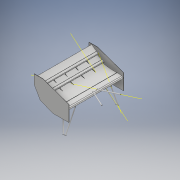
# Autodesk Inventor part: simpleRrwing
Saved by Autodesk Inventor 2018.2 (Build 222227000, 227)
## iProperties
Created: 2018-05-20
Part Number: simpleRrwing
Material: 一般
Document SubType Name: Modeling
Designer: ku_sk
Density: 1 g/cm^3
Appearance: 既定
Author: ku_sk
Autodesk Inventor part; units mm, degrees
ref_plane "YZ Plane" through (0, 0, 0) normal (1, 0, 0) x (0, 1, 0)
ref_plane "XZ Plane" through (0, 0, 0) normal (0, 1, 0) x (-1, 0, 0)
ref_plane "XY Plane" through (0, 0, 0) normal (0, 0, 1) x (1, 0, 0)
ref_plane "作業平面7" through (-254.1154, 478, -190) normal (0, 1, 0) x (1, 0, 0)
sketch "スケッチ4" plane through (-254.1154, 478, -190) normal (0, 1, 0) x (1, 0, 0)
  line L0 (-220, -86.6025) -> (0, 0) projected
  line L1 (-220, -86.6025) -> (-325.8846, -270) projected
  line L2 (-325.8846, -270) -> (-325.8846, -430) projected
  line L3 (-325.8846, -430) -> (-175.8846, -430) projected
  line L4 (-175.8846, -430) -> (274.1154, -270) projected
  line L5 (274.1154, -270) -> (274.1154, 0) projected
  line L6 (274.1154, 0) -> (0, 0) projected
  circle A0 centre (-165.8846, -335) radius 2.5 projected
  circle A1 centre (-65.8846, -265) radius 2.5 projected
  circle A2 centre (254.1154, -190) radius 2.5 projected
  point P0 (254.1154, -190)
extrude "押し出し1" add sketch "スケッチ4" against normal blind 5 contours L0 L6 L5 L4 L3 L2 L1 | A0 | A1 | A2
ref_plane "作業平面8" through (-254.1154, 473, -190) normal (0, -1, 0) x (1, 0, 0)
sketch "スケッチ5" plane through (-254.1154, 473, -190) normal (0, -1, 0) x (1, 0, 0)
  arc A0 (-98.825, 235.4012) -> (58.0734, 177.1204) centre (363.8757, 1240.7077) ccw projected
  arc A1 (-96.151, 242.9074) -> (-98.825, 235.4012) centre (-97.1526, 239.0348) ccw projected
  arc A2 (-96.151, 242.9074) -> (158.3312, 216.8528) centre (116.6772, 1065.8316) ccw projected
  arc A3 (158.3312, 216.8528) -> (163.3213, 217.108) centre (99.5256, 1415.411) ccw projected
  arc A4 (242.3807, 210.8189) -> (163.3213, 217.108) centre (179.2702, -82.4677) ccw projected
  arc A5 (262.2344, 202.6128) -> (242.3807, 210.8189) centre (229.7586, 152.1616) ccw projected
  arc A6 (263.5157, 178.3109) -> (262.2344, 202.6128) centre (254.1154, 190) ccw projected
  arc A7 (246.2233, 168.6632) -> (263.5157, 178.3109) centre (226.4942, 224.3463) ccw projected
  arc A8 (191.5251, 157.8735) -> (246.2233, 168.6632) centre (182.1223, 349.5809) ccw projected
  arc A9 (103.8035, 165.4256) -> (191.5251, 157.8735) centre (175.4883, 484.8376) ccw projected
  arc A10 (58.0734, 177.1204) -> (103.8035, 165.4256) centre (278.4325, 943.5344) ccw projected
  arc A11 (-197.55, 319.0808) -> (-142.9628, 280.3195) centre (85.3008, 659.5991) ccw projected
  arc A12 (-195.7398, 321.7041) -> (-197.55, 319.0808) centre (-196.5276, 320.3115) ccw projected
  arc A13 (-195.7398, 321.7041) -> (-100.1128, 285.2914) centre (-28.3139, 617.624) ccw projected
  arc A14 (-100.1128, 285.2914) -> (-98.1583, 284.8734) centre (1.2504, 754.4668) ccw projected
  arc A15 (-68.2632, 274.2587) -> (-98.1583, 284.8734) centre (-123.0105, 167.4751) ccw projected
  arc A16 (-61.4419, 269.0327) -> (-68.2632, 274.2587) centre (-79.2127, 252.902) ccw projected
  arc A17 (-63.4627, 259.5105) -> (-61.4419, 269.0327) centre (-65.8846, 265) ccw projected
  arc A18 (-71.1428, 257.5731) -> (-63.4627, 259.5105) centre (-73.0008, 281.13) ccw projected
  arc A19 (-93.3936, 259.0671) -> (-71.1428, 257.5731) centre (-77.1795, 334.1106) ccw projected
  arc A20 (-126.5048, 271.0666) -> (-93.3936, 259.0671) centre (-65.7399, 387.0566) ccw projected
  arc A21 (-142.9628, 280.3195) -> (-126.5048, 271.0666) centre (21.5225, 553.6259) ccw projected
  arc A22 (-279.0665, 421.3155) -> (-236.3714, 369.7468) centre (82.279, 677.0238) ccw projected
  arc A23 (-276.6389, 423.381) -> (-279.0665, 421.3155) centre (-277.7604, 422.2398) ccw projected
  arc A24 (-276.6389, 423.381) -> (-193.6946, 363.4589) centre (-38.3283, 665.8846) ccw projected
  arc A25 (-193.6946, 363.4589) -> (-191.915, 362.5493) centre (25.6461, 790.4128) ccw projected
  arc A26 (-165.7858, 344.5588) -> (-191.915, 362.5493) centre (-246.3053, 255.5835) ccw projected
  arc A27 (-160.5495, 337.7454) -> (-165.7858, 344.5588) centre (-181.8897, 326.7638) ccw projected
  arc A28 (-164.966, 329.0707) -> (-160.5495, 337.7454) centre (-165.8846, 335) ccw projected
  arc A29 (-172.8859, 329.1871) -> (-164.966, 329.0707) centre (-168.5836, 352.4222) ccw projected
  arc A30 (-193.9918, 336.3891) -> (-172.8859, 329.1871) centre (-158.9075, 404.679) ccw projected
  arc A31 (-222.869, 356.5496) -> (-193.9918, 336.3891) centre (-134.1543, 452.8602) ccw projected
  arc A32 (-236.3714, 369.7468) -> (-222.869, 356.5496) centre (-6.754, 591.1686) ccw projected
  point P0 (254.1154, 190)
extrude "押し出し2" add sketch "スケッチ5" along normal blind 186
sketch "スケッチ6" plane through (-254.1154, 287, -190) normal (0, -1, 0) x (1, 0, 0)
  arc A0 (-197.1682, 321.7777) -> (-197.55, 319.0808) centre (-196.5276, 320.3115) ccw projected
  arc A1 (-197.55, 319.0808) -> (-142.9628, 280.3195) centre (85.3008, 659.5991) ccw projected
  arc A2 (-142.9628, 280.3195) -> (-126.5048, 271.0666) centre (21.5225, 553.6259) ccw projected
  line L0 (-126.5048, 271.0666) -> (-94.3475, 254.22) projected
  arc A3 (-93.447, 249.6278) -> (-94.3475, 254.22) centre (-95.7396, 251.5626) ccw projected
  line L1 (-93.447, 249.6278) -> (-100.2095, 241.6146) projected
  arc A4 (-100.2095, 241.6146) -> (-98.825, 235.4012) centre (-97.1526, 239.0348) ccw projected
  arc A5 (-98.825, 235.4012) -> (58.0734, 177.1204) centre (363.8757, 1240.7077) ccw projected
  arc A6 (58.0734, 177.1204) -> (103.8035, 165.4256) centre (278.4325, 943.5344) ccw projected
  arc A7 (103.8035, 165.4256) -> (191.5251, 157.8735) centre (175.4883, 484.8376) ccw projected
  arc A8 (191.5251, 157.8735) -> (246.2233, 168.6632) centre (182.1223, 349.5809) ccw projected
  arc A9 (246.2233, 168.6632) -> (263.5157, 178.3109) centre (226.4942, 224.3463) ccw projected
  arc A10 (263.5157, 178.3109) -> (262.2344, 202.6128) centre (254.1154, 190) ccw projected
  arc A11 (262.2344, 202.6128) -> (242.3807, 210.8189) centre (229.7586, 152.1616) ccw projected
  arc A12 (242.3807, 210.8189) -> (163.3213, 217.108) centre (179.2702, -82.4677) ccw projected
  arc A13 (158.3312, 216.8528) -> (163.3213, 217.108) centre (99.5256, 1415.411) ccw projected
  arc A14 (-23.7761, 227.5161) -> (158.3312, 216.8528) centre (116.6772, 1065.8316) ccw projected
  arc A15 (-33.5904, 230.2106) -> (-23.7761, 227.5161) centre (-15.5142, 276.8287) ccw projected
  line L2 (-33.5904, 230.2106) -> (-75.8322, 246.5899) projected
  arc A16 (-76.0007, 253.979) -> (-75.8322, 246.5899) centre (-74.3861, 250.3193) ccw projected
  line L3 (-76.0007, 253.979) -> (-63.4627, 259.5105) projected
  arc A17 (-63.4627, 259.5105) -> (-61.4419, 269.0327) centre (-65.8846, 265) ccw projected
  arc A18 (-61.4419, 269.0327) -> (-68.2632, 274.2587) centre (-79.2127, 252.902) ccw projected
  arc A19 (-68.2632, 274.2587) -> (-98.1583, 284.8734) centre (-123.0105, 167.4751) ccw projected
  arc A20 (-100.1128, 285.2914) -> (-98.1583, 284.8734) centre (1.2504, 754.4668) ccw projected
  arc A21 (-133.4564, 294.2897) -> (-100.1128, 285.2914) centre (-28.3139, 617.624) ccw projected
  arc A22 (-147.5202, 301.4877) -> (-133.4564, 294.2897) centre (-117.9943, 341.8389) ccw projected
  line L4 (-147.5202, 301.4877) -> (-173.8847, 320.7792) projected
  arc A23 (-172.135, 327.9601) -> (-173.8847, 320.7792) centre (-171.5226, 324.0073) ccw projected
  line L5 (-172.135, 327.9601) -> (-164.966, 329.0707) projected
  arc A24 (-164.966, 329.0707) -> (-160.5495, 337.7454) centre (-165.8846, 335) ccw projected
  arc A25 (-160.5495, 337.7454) -> (-165.7858, 344.5588) centre (-181.8897, 326.7638) ccw projected
  arc A26 (-165.7858, 344.5588) -> (-191.915, 362.5493) centre (-246.3053, 255.5835) ccw projected
  arc A27 (-193.6946, 363.4589) -> (-191.915, 362.5493) centre (25.6461, 790.4128) ccw projected
  arc A28 (-276.6389, 423.381) -> (-193.6946, 363.4589) centre (-38.3283, 665.8846) ccw projected
  arc A29 (-276.6389, 423.381) -> (-279.0665, 421.3155) centre (-277.7604, 422.2398) ccw projected
  arc A30 (-279.0665, 421.3155) -> (-236.3714, 369.7468) centre (82.279, 677.0238) ccw projected
  arc A31 (-236.3714, 369.7468) -> (-222.869, 356.5496) centre (-6.754, 591.1686) ccw projected
  line L6 (-222.869, 356.5496) -> (-192.3777, 328.463) projected
  arc A32 (-193.2092, 323.5074) -> (-192.3777, 328.463) centre (-194.4102, 326.2565) ccw projected
  line L7 (-193.2092, 323.5074) -> (-197.1682, 321.7777) projected
  point P0 (254.1154, 190)
extrude "押し出し3" add sketch "スケッチ6" along normal blind 4
sketch "スケッチ7" plane through (-254.1154, 283, -190) normal (0, -1, 0) x (1, 0, 0)
  arc A0 (-98.825, 235.4012) -> (58.0734, 177.1204) centre (363.8757, 1240.7077) ccw
  arc A1 (-96.151, 242.9074) -> (-98.825, 235.4012) centre (-97.1526, 239.0348) ccw
  arc A2 (-96.151, 242.9074) -> (158.3312, 216.8528) centre (116.6772, 1065.8316) ccw
  arc A3 (158.3312, 216.8528) -> (163.3213, 217.108) centre (99.5256, 1415.411) ccw
  arc A4 (242.3807, 210.8189) -> (163.3213, 217.108) centre (179.2702, -82.4677) ccw
  arc A5 (262.2344, 202.6128) -> (242.3807, 210.8189) centre (229.7586, 152.1616) ccw
  arc A6 (263.5157, 178.3109) -> (262.2344, 202.6128) centre (254.1154, 190) ccw
  arc A7 (246.2233, 168.6632) -> (263.5157, 178.3109) centre (226.4942, 224.3463) ccw
  arc A8 (191.5251, 157.8735) -> (246.2233, 168.6632) centre (182.1223, 349.5809) ccw
  arc A9 (103.8035, 165.4256) -> (191.5251, 157.8735) centre (175.4883, 484.8376) ccw
  arc A10 (58.0734, 177.1204) -> (103.8035, 165.4256) centre (278.4325, 943.5344) ccw
  arc A11 (-197.55, 319.0808) -> (-142.9628, 280.3195) centre (85.3008, 659.5991) ccw
  arc A12 (-195.7398, 321.7041) -> (-197.55, 319.0808) centre (-196.5276, 320.3115) ccw
  arc A13 (-195.7398, 321.7041) -> (-100.1128, 285.2914) centre (-28.3139, 617.624) ccw
  arc A14 (-100.1128, 285.2914) -> (-98.1583, 284.8734) centre (1.2504, 754.4668) ccw
  arc A15 (-68.2632, 274.2587) -> (-98.1583, 284.8734) centre (-123.0105, 167.4751) ccw
  arc A16 (-61.4419, 269.0327) -> (-68.2632, 274.2587) centre (-79.2127, 252.902) ccw
  arc A17 (-63.4627, 259.5105) -> (-61.4419, 269.0327) centre (-65.8846, 265) ccw
  arc A18 (-71.1428, 257.5731) -> (-63.4627, 259.5105) centre (-73.0008, 281.13) ccw
  arc A19 (-93.3936, 259.0671) -> (-71.1428, 257.5731) centre (-77.1795, 334.1106) ccw
  arc A20 (-126.5048, 271.0666) -> (-93.3936, 259.0671) centre (-65.7399, 387.0566) ccw
  arc A21 (-142.9628, 280.3195) -> (-126.5048, 271.0666) centre (21.5225, 553.6259) ccw
  arc A22 (-279.0665, 421.3155) -> (-236.3714, 369.7468) centre (82.279, 677.0238) ccw
  arc A23 (-276.6389, 423.381) -> (-279.0665, 421.3155) centre (-277.7604, 422.2398) ccw
  arc A24 (-276.6389, 423.381) -> (-193.6946, 363.4589) centre (-38.3283, 665.8846) ccw
  arc A25 (-193.6946, 363.4589) -> (-191.915, 362.5493) centre (25.6461, 790.4128) ccw
  arc A26 (-165.7858, 344.5588) -> (-191.915, 362.5493) centre (-246.3053, 255.5835) ccw
  arc A27 (-160.5495, 337.7454) -> (-165.7858, 344.5588) centre (-181.8897, 326.7638) ccw
  arc A28 (-164.966, 329.0707) -> (-160.5495, 337.7454) centre (-165.8846, 335) ccw
  arc A29 (-172.8859, 329.1871) -> (-164.966, 329.0707) centre (-168.5836, 352.4222) ccw
  arc A30 (-193.9918, 336.3891) -> (-172.8859, 329.1871) centre (-158.9075, 404.679) ccw
  arc A31 (-222.869, 356.5496) -> (-193.9918, 336.3891) centre (-134.1543, 452.8602) ccw
  arc A32 (-236.3714, 369.7468) -> (-222.869, 356.5496) centre (-6.754, 591.1686) ccw
  point P0 (254.1154, 190)
  point P1 (254.1154, 190)
  constraints: 66 point on circle, 33 centre point
extrude "押し出し4" add sketch "スケッチ7" along normal blind 186
sketch "スケッチ8" plane through (-254.1154, 97, -190) normal (0, -1, 0) x (1, 0, 0)
  arc A0 (-197.1682, 321.7777) -> (-197.55, 319.0808) centre (-196.5276, 320.3115) ccw
  arc A1 (-197.55, 319.0808) -> (-142.9628, 280.3195) centre (85.3008, 659.5991) ccw
  arc A2 (-142.9628, 280.3195) -> (-126.5048, 271.0666) centre (21.5225, 553.6259) ccw
  line L0 (-126.5048, 271.0666) -> (-94.3475, 254.22)
  arc A3 (-93.447, 249.6278) -> (-94.3475, 254.22) centre (-95.7396, 251.5626) ccw
  line L1 (-93.447, 249.6278) -> (-100.2095, 241.6146)
  arc A4 (-100.2095, 241.6146) -> (-98.825, 235.4012) centre (-97.1526, 239.0348) ccw
  arc A5 (-98.825, 235.4012) -> (58.0734, 177.1204) centre (363.8757, 1240.7077) ccw
  arc A6 (58.0734, 177.1204) -> (103.8035, 165.4256) centre (278.4325, 943.5344) ccw
  arc A7 (103.8035, 165.4256) -> (191.5251, 157.8735) centre (175.4883, 484.8376) ccw
  arc A8 (191.5251, 157.8735) -> (246.2233, 168.6632) centre (182.1223, 349.5809) ccw
  arc A9 (246.2233, 168.6632) -> (263.5157, 178.3109) centre (226.4942, 224.3463) ccw
  arc A10 (263.5157, 178.3109) -> (262.2344, 202.6128) centre (254.1154, 190) ccw
  arc A11 (262.2344, 202.6128) -> (242.3807, 210.8189) centre (229.7586, 152.1616) ccw
  arc A12 (242.3807, 210.8189) -> (163.3213, 217.108) centre (179.2702, -82.4677) ccw
  arc A13 (158.3312, 216.8528) -> (163.3213, 217.108) centre (99.5256, 1415.411) ccw
  arc A14 (-23.7761, 227.5161) -> (158.3312, 216.8528) centre (116.6772, 1065.8316) ccw
  arc A15 (-33.5904, 230.2106) -> (-23.7761, 227.5161) centre (-15.5142, 276.8287) ccw
  line L2 (-33.5904, 230.2106) -> (-75.8322, 246.5899)
  arc A16 (-76.0007, 253.979) -> (-75.8322, 246.5899) centre (-74.3861, 250.3193) ccw
  line L3 (-76.0007, 253.979) -> (-63.4627, 259.5105)
  arc A17 (-63.4627, 259.5105) -> (-61.4419, 269.0327) centre (-65.8846, 265) ccw
  arc A18 (-61.4419, 269.0327) -> (-68.2632, 274.2587) centre (-79.2127, 252.902) ccw
  arc A19 (-68.2632, 274.2587) -> (-98.1583, 284.8734) centre (-123.0105, 167.4751) ccw
  arc A20 (-100.1128, 285.2914) -> (-98.1583, 284.8734) centre (1.2504, 754.4668) ccw
  arc A21 (-133.4564, 294.2897) -> (-100.1128, 285.2914) centre (-28.3139, 617.624) ccw
  arc A22 (-147.5202, 301.4877) -> (-133.4564, 294.2897) centre (-117.9943, 341.8389) ccw
  line L4 (-147.5202, 301.4877) -> (-173.8847, 320.7792)
  arc A23 (-172.135, 327.9601) -> (-173.8847, 320.7792) centre (-171.5226, 324.0073) ccw
  line L5 (-172.135, 327.9601) -> (-164.966, 329.0707)
  arc A24 (-164.966, 329.0707) -> (-160.5495, 337.7454) centre (-165.8846, 335) ccw
  arc A25 (-160.5495, 337.7454) -> (-165.7858, 344.5588) centre (-181.8897, 326.7638) ccw
  arc A26 (-165.7858, 344.5588) -> (-191.915, 362.5493) centre (-246.3053, 255.5835) ccw
  arc A27 (-193.6946, 363.4589) -> (-191.915, 362.5493) centre (25.6461, 790.4128) ccw
  arc A28 (-276.6389, 423.381) -> (-193.6946, 363.4589) centre (-38.3283, 665.8846) ccw
  arc A29 (-276.6389, 423.381) -> (-279.0665, 421.3155) centre (-277.7604, 422.2398) ccw
  arc A30 (-279.0665, 421.3155) -> (-236.3714, 369.7468) centre (82.279, 677.0238) ccw
  arc A31 (-236.3714, 369.7468) -> (-222.869, 356.5496) centre (-6.754, 591.1686) ccw
  line L6 (-222.869, 356.5496) -> (-192.3777, 328.463)
  arc A32 (-193.2092, 323.5074) -> (-192.3777, 328.463) centre (-194.4102, 326.2565) ccw
  line L7 (-193.2092, 323.5074) -> (-197.1682, 321.7777)
  point P0 (254.1154, 190)
  point P1 (254.1154, 190)
  constraints: 66 point on circle, 33 centre point, 16 end point
extrude "押し出し5" add sketch "スケッチ8" along normal blind 4
sketch "スケッチ9" plane through (-254.1154, 93, -190) normal (0, -1, 0) x (1, 0, 0)
  arc A0 (-98.825, 235.4012) -> (58.0734, 177.1204) centre (363.8757, 1240.7077) ccw
  arc A1 (-96.151, 242.9074) -> (-98.825, 235.4012) centre (-97.1526, 239.0348) ccw
  arc A2 (-96.151, 242.9074) -> (158.3312, 216.8528) centre (116.6772, 1065.8316) ccw
  arc A3 (158.3312, 216.8528) -> (163.3213, 217.108) centre (99.5256, 1415.411) ccw
  arc A4 (242.3807, 210.8189) -> (163.3213, 217.108) centre (179.2702, -82.4677) ccw
  arc A5 (262.2344, 202.6128) -> (242.3807, 210.8189) centre (229.7586, 152.1616) ccw
  arc A6 (263.5157, 178.3109) -> (262.2344, 202.6128) centre (254.1154, 190) ccw
  arc A7 (246.2233, 168.6632) -> (263.5157, 178.3109) centre (226.4942, 224.3463) ccw
  arc A8 (191.5251, 157.8735) -> (246.2233, 168.6632) centre (182.1223, 349.5809) ccw
  arc A9 (103.8035, 165.4256) -> (191.5251, 157.8735) centre (175.4883, 484.8376) ccw
  arc A10 (58.0734, 177.1204) -> (103.8035, 165.4256) centre (278.4325, 943.5344) ccw
  arc A11 (-197.55, 319.0808) -> (-142.9628, 280.3195) centre (85.3008, 659.5991) ccw
  arc A12 (-195.7398, 321.7041) -> (-197.55, 319.0808) centre (-196.5276, 320.3115) ccw
  arc A13 (-195.7398, 321.7041) -> (-100.1128, 285.2914) centre (-28.3139, 617.624) ccw
  arc A14 (-100.1128, 285.2914) -> (-98.1583, 284.8734) centre (1.2504, 754.4668) ccw
  arc A15 (-68.2632, 274.2587) -> (-98.1583, 284.8734) centre (-123.0105, 167.4751) ccw
  arc A16 (-61.4419, 269.0327) -> (-68.2632, 274.2587) centre (-79.2127, 252.902) ccw
  arc A17 (-63.4627, 259.5105) -> (-61.4419, 269.0327) centre (-65.8846, 265) ccw
  arc A18 (-71.1428, 257.5731) -> (-63.4627, 259.5105) centre (-73.0008, 281.13) ccw
  arc A19 (-93.3936, 259.0671) -> (-71.1428, 257.5731) centre (-77.1795, 334.1106) ccw
  arc A20 (-126.5048, 271.0666) -> (-93.3936, 259.0671) centre (-65.7399, 387.0566) ccw
  arc A21 (-142.9628, 280.3195) -> (-126.5048, 271.0666) centre (21.5225, 553.6259) ccw
  arc A22 (-279.0665, 421.3155) -> (-236.3714, 369.7468) centre (82.279, 677.0238) ccw
  arc A23 (-276.6389, 423.381) -> (-279.0665, 421.3155) centre (-277.7604, 422.2398) ccw
  arc A24 (-276.6389, 423.381) -> (-193.6946, 363.4589) centre (-38.3283, 665.8846) ccw
  arc A25 (-193.6946, 363.4589) -> (-191.915, 362.5493) centre (25.6461, 790.4128) ccw
  arc A26 (-165.7858, 344.5588) -> (-191.915, 362.5493) centre (-246.3053, 255.5835) ccw
  arc A27 (-160.5495, 337.7454) -> (-165.7858, 344.5588) centre (-181.8897, 326.7638) ccw
  arc A28 (-164.966, 329.0707) -> (-160.5495, 337.7454) centre (-165.8846, 335) ccw
  arc A29 (-172.8859, 329.1871) -> (-164.966, 329.0707) centre (-168.5836, 352.4222) ccw
  arc A30 (-193.9918, 336.3891) -> (-172.8859, 329.1871) centre (-158.9075, 404.679) ccw
  arc A31 (-222.869, 356.5496) -> (-193.9918, 336.3891) centre (-134.1543, 452.8602) ccw
  arc A32 (-236.3714, 369.7468) -> (-222.869, 356.5496) centre (-6.754, 591.1686) ccw
  point P0 (254.1154, 190)
  point P1 (254.1154, 190)
  constraints: 66 point on circle, 33 centre point
extrude "押し出し6" add sketch "スケッチ9" along normal blind 186
sketch "スケッチ10" plane through (-254.1154, -93, -190) normal (0, -1, 0) x (1, 0, 0)
  arc A0 (-197.1682, 321.7777) -> (-197.55, 319.0808) centre (-196.5276, 320.3115) ccw
  arc A1 (-197.55, 319.0808) -> (-142.9628, 280.3195) centre (85.3008, 659.5991) ccw
  arc A2 (-142.9628, 280.3195) -> (-126.5048, 271.0666) centre (21.5225, 553.6259) ccw
  line L0 (-126.5048, 271.0666) -> (-94.3475, 254.22)
  arc A3 (-93.447, 249.6278) -> (-94.3475, 254.22) centre (-95.7396, 251.5626) ccw
  line L1 (-93.447, 249.6278) -> (-100.2095, 241.6146)
  arc A4 (-100.2095, 241.6146) -> (-98.825, 235.4012) centre (-97.1526, 239.0348) ccw
  arc A5 (-98.825, 235.4012) -> (58.0734, 177.1204) centre (363.8757, 1240.7077) ccw
  arc A6 (58.0734, 177.1204) -> (103.8035, 165.4256) centre (278.4325, 943.5344) ccw
  arc A7 (103.8035, 165.4256) -> (191.5251, 157.8735) centre (175.4883, 484.8376) ccw
  arc A8 (191.5251, 157.8735) -> (246.2233, 168.6632) centre (182.1223, 349.5809) ccw
  arc A9 (246.2233, 168.6632) -> (263.5157, 178.3109) centre (226.4942, 224.3463) ccw
  arc A10 (263.5157, 178.3109) -> (262.2344, 202.6128) centre (254.1154, 190) ccw
  arc A11 (262.2344, 202.6128) -> (242.3807, 210.8189) centre (229.7586, 152.1616) ccw
  arc A12 (242.3807, 210.8189) -> (163.3213, 217.108) centre (179.2702, -82.4677) ccw
  arc A13 (158.3312, 216.8528) -> (163.3213, 217.108) centre (99.5256, 1415.411) ccw
  arc A14 (-23.7761, 227.5161) -> (158.3312, 216.8528) centre (116.6772, 1065.8316) ccw
  arc A15 (-33.5904, 230.2106) -> (-23.7761, 227.5161) centre (-15.5142, 276.8287) ccw
  line L2 (-33.5904, 230.2106) -> (-75.8322, 246.5899)
  arc A16 (-76.0007, 253.979) -> (-75.8322, 246.5899) centre (-74.3861, 250.3193) ccw
  line L3 (-76.0007, 253.979) -> (-63.4627, 259.5105)
  arc A17 (-63.4627, 259.5105) -> (-61.4419, 269.0327) centre (-65.8846, 265) ccw
  arc A18 (-61.4419, 269.0327) -> (-68.2632, 274.2587) centre (-79.2127, 252.902) ccw
  arc A19 (-68.2632, 274.2587) -> (-98.1583, 284.8734) centre (-123.0105, 167.4751) ccw
  arc A20 (-100.1128, 285.2914) -> (-98.1583, 284.8734) centre (1.2504, 754.4668) ccw
  arc A21 (-133.4564, 294.2897) -> (-100.1128, 285.2914) centre (-28.3139, 617.624) ccw
  arc A22 (-147.5202, 301.4877) -> (-133.4564, 294.2897) centre (-117.9943, 341.8389) ccw
  line L4 (-147.5202, 301.4877) -> (-173.8847, 320.7792)
  arc A23 (-172.135, 327.9601) -> (-173.8847, 320.7792) centre (-171.5226, 324.0073) ccw
  line L5 (-172.135, 327.9601) -> (-164.966, 329.0707)
  arc A24 (-164.966, 329.0707) -> (-160.5495, 337.7454) centre (-165.8846, 335) ccw
  arc A25 (-160.5495, 337.7454) -> (-165.7858, 344.5588) centre (-181.8897, 326.7638) ccw
  arc A26 (-165.7858, 344.5588) -> (-191.915, 362.5493) centre (-246.3053, 255.5835) ccw
  arc A27 (-193.6946, 363.4589) -> (-191.915, 362.5493) centre (25.6461, 790.4128) ccw
  arc A28 (-276.6389, 423.381) -> (-193.6946, 363.4589) centre (-38.3283, 665.8846) ccw
  arc A29 (-276.6389, 423.381) -> (-279.0665, 421.3155) centre (-277.7604, 422.2398) ccw
  arc A30 (-279.0665, 421.3155) -> (-236.3714, 369.7468) centre (82.279, 677.0238) ccw
  arc A31 (-236.3714, 369.7468) -> (-222.869, 356.5496) centre (-6.754, 591.1686) ccw
  line L6 (-222.869, 356.5496) -> (-192.3777, 328.463)
  arc A32 (-193.2092, 323.5074) -> (-192.3777, 328.463) centre (-194.4102, 326.2565) ccw
  line L7 (-193.2092, 323.5074) -> (-197.1682, 321.7777)
  point P0 (254.1154, 190)
  point P1 (254.1154, 190)
  point P2 (254.1154, 190)
  constraints: 66 point on circle, 33 centre point, 16 end point
extrude "押し出し7" add sketch "スケッチ10" along normal blind 4
sketch "スケッチ11" plane through (-254.1154, -97, -190) normal (0, -1, 0) x (1, 0, 0)
  arc A0 (-98.825, 235.4012) -> (58.0734, 177.1204) centre (363.8757, 1240.7077) ccw
  arc A1 (-96.151, 242.9074) -> (-98.825, 235.4012) centre (-97.1526, 239.0348) ccw
  arc A2 (-96.151, 242.9074) -> (158.3312, 216.8528) centre (116.6772, 1065.8316) ccw
  arc A3 (158.3312, 216.8528) -> (163.3213, 217.108) centre (99.5256, 1415.411) ccw
  arc A4 (242.3807, 210.8189) -> (163.3213, 217.108) centre (179.2702, -82.4677) ccw
  arc A5 (262.2344, 202.6128) -> (242.3807, 210.8189) centre (229.7586, 152.1616) ccw
  arc A6 (263.5157, 178.3109) -> (262.2344, 202.6128) centre (254.1154, 190) ccw
  arc A7 (246.2233, 168.6632) -> (263.5157, 178.3109) centre (226.4942, 224.3463) ccw
  arc A8 (191.5251, 157.8735) -> (246.2233, 168.6632) centre (182.1223, 349.5809) ccw
  arc A9 (103.8035, 165.4256) -> (191.5251, 157.8735) centre (175.4883, 484.8376) ccw
  arc A10 (58.0734, 177.1204) -> (103.8035, 165.4256) centre (278.4325, 943.5344) ccw
  arc A11 (-197.55, 319.0808) -> (-142.9628, 280.3195) centre (85.3008, 659.5991) ccw
  arc A12 (-195.7398, 321.7041) -> (-197.55, 319.0808) centre (-196.5276, 320.3115) ccw
  arc A13 (-195.7398, 321.7041) -> (-100.1128, 285.2914) centre (-28.3139, 617.624) ccw
  arc A14 (-100.1128, 285.2914) -> (-98.1583, 284.8734) centre (1.2504, 754.4668) ccw
  arc A15 (-68.2632, 274.2587) -> (-98.1583, 284.8734) centre (-123.0105, 167.4751) ccw
  arc A16 (-61.4419, 269.0327) -> (-68.2632, 274.2587) centre (-79.2127, 252.902) ccw
  arc A17 (-63.4627, 259.5105) -> (-61.4419, 269.0327) centre (-65.8846, 265) ccw
  arc A18 (-71.1428, 257.5731) -> (-63.4627, 259.5105) centre (-73.0008, 281.13) ccw
  arc A19 (-93.3936, 259.0671) -> (-71.1428, 257.5731) centre (-77.1795, 334.1106) ccw
  arc A20 (-126.5048, 271.0666) -> (-93.3936, 259.0671) centre (-65.7399, 387.0566) ccw
  arc A21 (-142.9628, 280.3195) -> (-126.5048, 271.0666) centre (21.5225, 553.6259) ccw
  arc A22 (-279.0665, 421.3155) -> (-236.3714, 369.7468) centre (82.279, 677.0238) ccw
  arc A23 (-276.6389, 423.381) -> (-279.0665, 421.3155) centre (-277.7604, 422.2398) ccw
  arc A24 (-276.6389, 423.381) -> (-193.6946, 363.4589) centre (-38.3283, 665.8846) ccw
  arc A25 (-193.6946, 363.4589) -> (-191.915, 362.5493) centre (25.6461, 790.4128) ccw
  arc A26 (-165.7858, 344.5588) -> (-191.915, 362.5493) centre (-246.3053, 255.5835) ccw
  arc A27 (-160.5495, 337.7454) -> (-165.7858, 344.5588) centre (-181.8897, 326.7638) ccw
  arc A28 (-164.966, 329.0707) -> (-160.5495, 337.7454) centre (-165.8846, 335) ccw
  arc A29 (-172.8859, 329.1871) -> (-164.966, 329.0707) centre (-168.5836, 352.4222) ccw
  arc A30 (-193.9918, 336.3891) -> (-172.8859, 329.1871) centre (-158.9075, 404.679) ccw
  arc A31 (-222.869, 356.5496) -> (-193.9918, 336.3891) centre (-134.1543, 452.8602) ccw
  arc A32 (-236.3714, 369.7468) -> (-222.869, 356.5496) centre (-6.754, 591.1686) ccw
  point P0 (254.1154, 190)
  point P1 (254.1154, 190)
  point P2 (254.1154, 190)
  constraints: 66 point on circle, 33 centre point
extrude "押し出し8" add sketch "スケッチ11" along normal blind 186
sketch "スケッチ12" plane through (-254.1154, -283, -190) normal (0, -1, 0) x (1, 0, 0)
  arc A0 (-197.1682, 321.7777) -> (-197.55, 319.0808) centre (-196.5276, 320.3115) ccw
  arc A1 (-197.55, 319.0808) -> (-142.9628, 280.3195) centre (85.3008, 659.5991) ccw
  arc A2 (-142.9628, 280.3195) -> (-126.5048, 271.0666) centre (21.5225, 553.6259) ccw
  line L0 (-126.5048, 271.0666) -> (-94.3475, 254.22)
  arc A3 (-93.447, 249.6278) -> (-94.3475, 254.22) centre (-95.7396, 251.5626) ccw
  line L1 (-93.447, 249.6278) -> (-100.2095, 241.6146)
  arc A4 (-100.2095, 241.6146) -> (-98.825, 235.4012) centre (-97.1526, 239.0348) ccw
  arc A5 (-98.825, 235.4012) -> (58.0734, 177.1204) centre (363.8757, 1240.7077) ccw
  arc A6 (58.0734, 177.1204) -> (103.8035, 165.4256) centre (278.4325, 943.5344) ccw
  arc A7 (103.8035, 165.4256) -> (191.5251, 157.8735) centre (175.4883, 484.8376) ccw
  arc A8 (191.5251, 157.8735) -> (246.2233, 168.6632) centre (182.1223, 349.5809) ccw
  arc A9 (246.2233, 168.6632) -> (263.5157, 178.3109) centre (226.4942, 224.3463) ccw
  arc A10 (263.5157, 178.3109) -> (262.2344, 202.6128) centre (254.1154, 190) ccw
  arc A11 (262.2344, 202.6128) -> (242.3807, 210.8189) centre (229.7586, 152.1616) ccw
  arc A12 (242.3807, 210.8189) -> (163.3213, 217.108) centre (179.2702, -82.4677) ccw
  arc A13 (158.3312, 216.8528) -> (163.3213, 217.108) centre (99.5256, 1415.411) ccw
  arc A14 (-23.7761, 227.5161) -> (158.3312, 216.8528) centre (116.6772, 1065.8316) ccw
  arc A15 (-33.5904, 230.2106) -> (-23.7761, 227.5161) centre (-15.5142, 276.8287) ccw
  line L2 (-33.5904, 230.2106) -> (-75.8322, 246.5899)
  arc A16 (-76.0007, 253.979) -> (-75.8322, 246.5899) centre (-74.3861, 250.3193) ccw
  line L3 (-76.0007, 253.979) -> (-63.4627, 259.5105)
  arc A17 (-63.4627, 259.5105) -> (-61.4419, 269.0327) centre (-65.8846, 265) ccw
  arc A18 (-61.4419, 269.0327) -> (-68.2632, 274.2587) centre (-79.2127, 252.902) ccw
  arc A19 (-68.2632, 274.2587) -> (-98.1583, 284.8734) centre (-123.0105, 167.4751) ccw
  arc A20 (-100.1128, 285.2914) -> (-98.1583, 284.8734) centre (1.2504, 754.4668) ccw
  arc A21 (-133.4564, 294.2897) -> (-100.1128, 285.2914) centre (-28.3139, 617.624) ccw
  arc A22 (-147.5202, 301.4877) -> (-133.4564, 294.2897) centre (-117.9943, 341.8389) ccw
  line L4 (-147.5202, 301.4877) -> (-173.8847, 320.7792)
  arc A23 (-172.135, 327.9601) -> (-173.8847, 320.7792) centre (-171.5226, 324.0073) ccw
  line L5 (-172.135, 327.9601) -> (-164.966, 329.0707)
  arc A24 (-164.966, 329.0707) -> (-160.5495, 337.7454) centre (-165.8846, 335) ccw
  arc A25 (-160.5495, 337.7454) -> (-165.7858, 344.5588) centre (-181.8897, 326.7638) ccw
  arc A26 (-165.7858, 344.5588) -> (-191.915, 362.5493) centre (-246.3053, 255.5835) ccw
  arc A27 (-193.6946, 363.4589) -> (-191.915, 362.5493) centre (25.6461, 790.4128) ccw
  arc A28 (-276.6389, 423.381) -> (-193.6946, 363.4589) centre (-38.3283, 665.8846) ccw
  arc A29 (-276.6389, 423.381) -> (-279.0665, 421.3155) centre (-277.7604, 422.2398) ccw
  arc A30 (-279.0665, 421.3155) -> (-236.3714, 369.7468) centre (82.279, 677.0238) ccw
  arc A31 (-236.3714, 369.7468) -> (-222.869, 356.5496) centre (-6.754, 591.1686) ccw
  line L6 (-222.869, 356.5496) -> (-192.3777, 328.463)
  arc A32 (-193.2092, 323.5074) -> (-192.3777, 328.463) centre (-194.4102, 326.2565) ccw
  line L7 (-193.2092, 323.5074) -> (-197.1682, 321.7777)
  point P0 (254.1154, 190)
  point P1 (254.1154, 190)
  point P2 (254.1154, 190)
  point P3 (254.1154, 190)
  constraints: 66 point on circle, 33 centre point, 16 end point
extrude "押し出し9" add sketch "スケッチ12" along normal blind 4
sketch "スケッチ13" plane through (-254.1154, -287, -190) normal (0, -1, 0) x (1, 0, 0)
  arc A0 (-98.825, 235.4012) -> (58.0734, 177.1204) centre (363.8757, 1240.7077) ccw
  arc A1 (-96.151, 242.9074) -> (-98.825, 235.4012) centre (-97.1526, 239.0348) ccw
  arc A2 (-96.151, 242.9074) -> (158.3312, 216.8528) centre (116.6772, 1065.8316) ccw
  arc A3 (158.3312, 216.8528) -> (163.3213, 217.108) centre (99.5256, 1415.411) ccw
  arc A4 (242.3807, 210.8189) -> (163.3213, 217.108) centre (179.2702, -82.4677) ccw
  arc A5 (262.2344, 202.6128) -> (242.3807, 210.8189) centre (229.7586, 152.1616) ccw
  arc A6 (263.5157, 178.3109) -> (262.2344, 202.6128) centre (254.1154, 190) ccw
  arc A7 (246.2233, 168.6632) -> (263.5157, 178.3109) centre (226.4942, 224.3463) ccw
  arc A8 (191.5251, 157.8735) -> (246.2233, 168.6632) centre (182.1223, 349.5809) ccw
  arc A9 (103.8035, 165.4256) -> (191.5251, 157.8735) centre (175.4883, 484.8376) ccw
  arc A10 (58.0734, 177.1204) -> (103.8035, 165.4256) centre (278.4325, 943.5344) ccw
  arc A11 (-197.55, 319.0808) -> (-142.9628, 280.3195) centre (85.3008, 659.5991) ccw
  arc A12 (-195.7398, 321.7041) -> (-197.55, 319.0808) centre (-196.5276, 320.3115) ccw
  arc A13 (-195.7398, 321.7041) -> (-100.1128, 285.2914) centre (-28.3139, 617.624) ccw
  arc A14 (-100.1128, 285.2914) -> (-98.1583, 284.8734) centre (1.2504, 754.4668) ccw
  arc A15 (-68.2632, 274.2587) -> (-98.1583, 284.8734) centre (-123.0105, 167.4751) ccw
  arc A16 (-61.4419, 269.0327) -> (-68.2632, 274.2587) centre (-79.2127, 252.902) ccw
  arc A17 (-63.4627, 259.5105) -> (-61.4419, 269.0327) centre (-65.8846, 265) ccw
  arc A18 (-71.1428, 257.5731) -> (-63.4627, 259.5105) centre (-73.0008, 281.13) ccw
  arc A19 (-93.3936, 259.0671) -> (-71.1428, 257.5731) centre (-77.1795, 334.1106) ccw
  arc A20 (-126.5048, 271.0666) -> (-93.3936, 259.0671) centre (-65.7399, 387.0566) ccw
  arc A21 (-142.9628, 280.3195) -> (-126.5048, 271.0666) centre (21.5225, 553.6259) ccw
  arc A22 (-279.0665, 421.3155) -> (-236.3714, 369.7468) centre (82.279, 677.0238) ccw
  arc A23 (-276.6389, 423.381) -> (-279.0665, 421.3155) centre (-277.7604, 422.2398) ccw
  arc A24 (-276.6389, 423.381) -> (-193.6946, 363.4589) centre (-38.3283, 665.8846) ccw
  arc A25 (-193.6946, 363.4589) -> (-191.915, 362.5493) centre (25.6461, 790.4128) ccw
  arc A26 (-165.7858, 344.5588) -> (-191.915, 362.5493) centre (-246.3053, 255.5835) ccw
  arc A27 (-160.5495, 337.7454) -> (-165.7858, 344.5588) centre (-181.8897, 326.7638) ccw
  arc A28 (-164.966, 329.0707) -> (-160.5495, 337.7454) centre (-165.8846, 335) ccw
  arc A29 (-172.8859, 329.1871) -> (-164.966, 329.0707) centre (-168.5836, 352.4222) ccw
  arc A30 (-193.9918, 336.3891) -> (-172.8859, 329.1871) centre (-158.9075, 404.679) ccw
  arc A31 (-222.869, 356.5496) -> (-193.9918, 336.3891) centre (-134.1543, 452.8602) ccw
  arc A32 (-236.3714, 369.7468) -> (-222.869, 356.5496) centre (-6.754, 591.1686) ccw
  point P0 (254.1154, 190)
  point P1 (254.1154, 190)
  point P2 (254.1154, 190)
  point P3 (254.1154, 190)
  constraints: 66 point on circle, 33 centre point
extrude "押し出し10" add sketch "スケッチ13" along normal blind 186
sketch "スケッチ14" plane through (-254.1154, -473, -190) normal (0, -1, 0) x (1, 0, 0)
  line L0 (0, 0) -> (-220, 86.6025) projected
  line L1 (0, 0) -> (274.1154, 0) projected
  line L2 (274.1154, 0) -> (274.1154, 270) projected
  line L3 (274.1154, 270) -> (-175.8846, 430) projected
  line L4 (-175.8846, 430) -> (-325.8846, 430) projected
  line L5 (-325.8846, 430) -> (-325.8846, 270) projected
  line L6 (-325.8846, 270) -> (-220, 86.6025) projected
  circle A0 centre (-165.8846, 335) radius 2.5 projected
  circle A1 centre (-65.8846, 265) radius 2.5 projected
  circle A2 centre (254.1154, 190) radius 2.5 projected
  point P0 (254.1154, 190)
extrude "押し出し11" add sketch "スケッチ14" along normal blind 5 contours L0 L6 L5 L4 L3 L2 L1 | A0 | A1 | A2
sketch "スケッチ16" plane through (0, 0, 0) normal (1, 0, 0) x (0, 1, 0)
  ellipse E0 centre (37.9281, 40.36) end of major axis (37.9233, 32.36) minor radius 7.2845 projected
  point P0 (0, 0)
  constraints: 1 other
sketch3d "3D スケッチ1"
  line L0 (-0.9802, 37.8986, 40.36) -> (279.3133, 165.1473, 40.2842)
sweep "スイープ1" add profiles "スケッチ16" path "3D スケッチ1"
ref_plane "作業平面5" through (-27.303, 313.7, -79.7865) normal (0, 0, -1) x (-1, 0, 0)
sketch "スケッチ18" plane through (-27.303, 313.7, -79.7865) normal (0, 0, -1) x (-1, 0, 0)
  ellipse E0 centre (7.5395, 2.7626) end of major axis (15.4422, 1.5191) minor radius 7.4166 projected
  point P0 (-27.303, -313.7)
  constraints: 1 other
sketch3d "3D スケッチ2"
  line L0 (-33.7855, 309.7452, -65.4182) -> (-56.8492, 456.3222, -432.3594)
sweep "スイープ2" add profiles "スケッチ18" path "3D スケッチ2"
ref_plane "作業平面6" through (-241.9696, 313.7, -47.8167) normal (0, 0, -1) x (-1, 0, 0)
sketch "スケッチ19" plane through (-241.9696, 313.7, -47.8167) normal (0, 0, -1) x (-1, 0, 0)
  ellipse E0 centre (-2.8511, -1.9312) end of major axis (-8.48, -7.6158) minor radius 7.061 projected
  point P0 (-241.9696, -313.7)
  constraints: 1 other
sketch3d "3D スケッチ3"
  line L0 (-241.7358, 309.1771, -32.9663) -> (-89.5884, 459.8319, -434.993)
sweep "スイープ3" add profiles "スケッチ19" path "3D スケッチ3"
mirror "ミラー1" about plane through (0, 0, 0) normal (0, 1, 0) of "スイープ1", "スイープ2", "スイープ3" bodies 2
